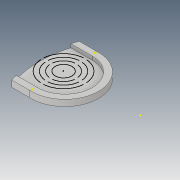
# Autodesk Inventor part: bottomThrusterCover
Saved by Autodesk Inventor 2018 (Build 220112000, 112)
## iProperties
Created: 2020-02-23
Part Number: bottomThrusterCover
Material: Generic
Document SubType Name: Modeling
Designer: anirudh
Density: 1 g/cm^3
Appearance: Default
Author: anirudh
Autodesk Inventor part; units mm, degrees
ref_plane "YZ Plane" through (0, 0, 0) normal (1, 0, 0) x (0, 1, 0)
ref_plane "XZ Plane" through (0, 0, 0) normal (0, 1, 0) x (-1, 0, 0)
ref_plane "XY Plane" through (0, 0, 0) normal (0, 0, 1) x (1, 0, 0)
sketch "Sketch1" plane through (0, 0, 0) normal (0, 1, 0) x (-1, 0, 0)
  circle A0 centre (155.3464, -63.5) radius 1.75
  circle A1 centre (155.3464, 63.5) radius 1.75
  arc A2 (195.546, -55.245) -> (195.546, 55.245) centre (0, 0) ccw
  circle A3 centre (155.3464, -63.5) radius 1.75
  circle A4 centre (155.3464, 63.5) radius 1.75
  arc A5 (191.5106, -67.9259) -> (191.5106, 67.9259) centre (0, 0) ccw
  arc A6 (155.758, 67.9259) -> (155.758, -67.9259) centre (152.4, 0) ccw
  line L0 (155.758, 67.9259) -> (191.5106, 67.9259)
  line L1 (155.758, -67.9259) -> (191.5106, -67.9259)
  point P0 (152.4, -50.8)
  point P1 (152.4, 50.8)
  point P2 (195.6623, -54.8317)
  constraints: 8 point on circle, 7 centre point, 4 end point, 2 concentric, 2 horizontal, 1 coincident
ref_plane "Work Plane2" through (0, 12.7, 0) normal (0, 1, 0) x (1, 0, 0)
sketch "Sketch3" plane through (0, 12.7, 0) normal (0, 1, 0) x (1, 0, 0)
  arc A0 (-155.758, -67.9259) -> (-155.758, 67.9259) centre (-152.4, 0) ccw projected
  arc A1 (-152.4, -55.245) -> (-152.4, 55.245) centre (-152.4, 0) ccw
  line L0 (-152.4, 55.245) -> (-195.546, 55.245)
  line L1 (-152.4, -55.245) -> (-195.546, -55.245)
  arc A2 (-191.5106, 67.9259) -> (-191.5106, -67.9259) centre (0, 0) ccw projected
  arc A3 (-195.546, 55.245) -> (-195.546, -55.245) centre (0, 0) ccw
  constraints: 5 point on circle, 4 end point, 2 centre point, 2 coincident, 2 horizontal
ref_plane "Work Plane3" through (0, 5.588, 0) normal (0, 1, 0) x (1, 0, 0)
ref_plane "Work Plane1" through (0, 12.7, 0) normal (0, 1, 0) x (1, 0, 0)
extrude "Extrusion6" add sketch "Sketch1" along normal blind 12.7
extrude "Extrusion7" cut sketch "Sketch3" against normal blind 7.112
sketch "Sketch6" plane through (0, 12.7, 0) normal (0, 1, 0) x (1, 0, 0)
  circle A0 centre (-155.3464, 63.5) radius 1.75 projected
  circle A1 centre (-155.3464, -63.5) radius 1.75 projected
  circle A2 centre (-155.3464, 0) radius 16.8275
  arc A3 (-129.8256, 3.175) -> (-152.1714, 25.5208) centre (-155.3464, 0) ccw
  arc A4 (-120.8848, 3.175) -> (-152.1714, 34.4616) centre (-155.3464, 0) ccw
  arc A5 (-152.1714, -25.5208) -> (-129.8256, -3.175) centre (-155.3464, 0) ccw
  arc A6 (-152.1714, -34.4616) -> (-120.8848, -3.175) centre (-155.3464, 0) ccw
  arc A7 (-158.5214, 25.5208) -> (-180.8672, 3.175) centre (-155.3464, 0) ccw
  arc A8 (-180.8672, -3.175) -> (-158.5214, -25.5208) centre (-155.3464, 0) ccw
  arc A9 (-158.5214, 34.4616) -> (-189.808, 3.175) centre (-155.3464, 0) ccw
  arc A10 (-189.808, -3.175) -> (-158.5214, -34.4616) centre (-155.3464, 0) ccw
  arc A11 (-158.5214, 43.3815) -> (-198.7279, 3.175) centre (-155.3464, 0) ccw
  arc A12 (-198.7279, -3.175) -> (-158.5214, -43.3815) centre (-155.3464, 0) ccw
  arc A13 (-152.1714, -43.3815) -> (-111.9649, -3.175) centre (-155.3464, 0) ccw
  arc A14 (-111.9649, 3.175) -> (-152.1714, 43.3815) centre (-155.3464, 0) ccw
  point P0 (0, 0)
  constraints: 24 point on circle, 13 centre point, 3 coincident
body "Solid3"
